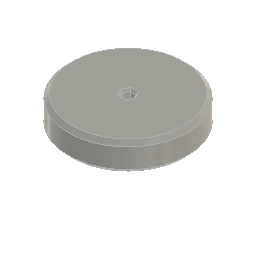
Assembly (Autodesk Fusion 360 archive; units mm, degrees)
design "Flywheel"
Autodesk Fusion 360 part; units mm, degrees
(part 1 of 2)
sketch "Sketch1" plane through (0, 0, 0) normal (0, 0, 1) x (1, 0, 0)
  circle A0 centre (0, 0) radius 2.5
  line L0 (1.3856, 0) -> (0.6928, 1.2)
  line L1 (0.6928, 1.2) -> (-0.6928, 1.2)
  line L2 (-0.6928, 1.2) -> (-1.3856, 0)
  line L3 (-1.3856, 0) -> (-0.6928, -1.2)
  line L4 (-0.6928, -1.2) -> (0.6928, -1.2)
  line L5 (0.6928, -1.2) -> (1.3856, 0)
  dimension "d2" = 5
  dimension "d11" = 2.4
  constraint coincident A0.centre origin
  constraint horizontal L1
  measures "d2" diameter of A0
  measures "d11" distance of L0 L3
extrude "Extrude1" add sketch "Sketch1" along normal blind 8
sketch "Sketch2" plane through (0, 0, 8) normal (0, 0, 1) x (-1, 0, 0)
  circle A0 centre (0, 0) radius 2.5
  circle A1 centre (0, 0) radius 15
  line L0 (-1.3856, 0) -> (-0.6928, 1.2)
  line L1 (-0.6928, 1.2) -> (0.6928, 1.2)
  line L2 (0.6928, 1.2) -> (1.3856, 0)
  line L3 (1.3856, 0) -> (0.6928, -1.2)
  line L4 (0.6928, -1.2) -> (-0.6928, -1.2)
  line L5 (-0.6928, -1.2) -> (-1.3856, 0)
  line L6 (0.6928, -1.2) -> (1.3856, 0)
  line L7 (1.3856, 0) -> (0.6928, 1.2)
  line L8 (0.6928, 1.2) -> (-0.6928, 1.2)
  line L9 (-0.6928, 1.2) -> (-1.3856, 0)
  line L10 (-1.3856, 0) -> (-0.6928, -1.2)
  line L11 (-0.6928, -1.2) -> (0.6928, -1.2)
  dimension "d5" = 30
  dimension "d12" = 2.4
  constraint coincident A0.centre A1.centre
  constraint horizontal L11
  measures "d5" diameter of A1
  measures "d12" distance of L8 L11
extrude "Extrude2" add sketch "Sketch2" along normal blind 7 contours A0 | A1
chamfer "Chamfer1" distance 0.5 angle 45 6 edges at (-1.0392, 0.6, 15) (-1.0392, -0.6, 15) (0, -1.2, 15) (1.0392, -0.6, 15) (1.0392, 0.6, 15) (0, 1.2, 15)
chamfer "Chamfer2" distance 1 angle 45 3 edges at (-2.3308, -0.904, 8) (13.9849, 5.4242, 8) (13.9849, 5.4242, 15)
chamfer "Chamfer3" distance 0.5 angle 45 6 edges at (1.0392, 0.6, 0) (0, 1.2, 0) (-1.0392, 0.6, 0) (-1.0392, -0.6, 0) (0, -1.2, 0) (1.0392, -0.6, 0)

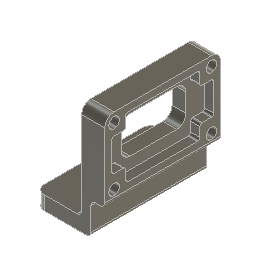
design "RPI Cam Mount"
Autodesk Fusion 360 part; units mm, degrees
sketch "Sketch1" plane through (0, 0, 0) normal (0, 0, 1) x (1, 0, 0)
  line L0 (0, 0) -> (-15, 0)
  line L1 (-15, 0) -> (-15, -25)
  line L2 (-15, -25) -> (0, -25)
  line L3 (0, -25) -> (0, 0)
  dimension "d1" = 15
  dimension "d2" = 25
  constraint horizontal L0
  constraint vertical L1
  constraint horizontal L2
  constraint vertical L3
  constraint coincident L0.start L3.end
  measures "d1" distance of L0.start L0.end
  measures "d2" distance of L0.end L1.end
extrude "Extrude1" add sketch "Sketch1" along normal blind 3
sketch "Sketch2" plane through (0, 0, 3) normal (0, 0, 1) x (-1, 0, 0)
  line L0 (0, 25) -> (0, 0)
  line L1 (0, 0) -> (15, 0)
  line L2 (15, 0) -> (15, 25)
  line L3 (15, 25) -> (0, 25)
  line L4 (0, 0) -> (5, 0)
  line L5 (5, 0) -> (5, 25)
  line L6 (5, 25) -> (0, 25)
  line L7 (0, 25) -> (0, 0)
  dimension "d5" = 5
  constraint horizontal L4
  constraint vertical L5
  constraint horizontal L6
  constraint vertical L7
  constraint coincident L3 L5.end
  constraint coincident L0.end L1.start
  measures "d5" distance of L0.end L4.end
extrude "Extrude2" add sketch "Sketch2" along normal blind 21 contours L0 L1 L3 L4 L5 L6 L7
sketch "Sketch3" plane through (0, 0, 0) normal (1, 0, 0) x (0, 1, 0)
  line L0 (-25, 0) -> (0, 0)
  line L1 (0, 0) -> (0, 24)
  line L2 (0, 24) -> (-25, 24)
  line L3 (-25, 24) -> (-25, 0)
  circle A0 centre (-23, 9.5) radius 1.15
  circle A1 centre (-23, 22) radius 1.15
  circle A2 centre (-2, 22) radius 1.15
  circle A3 centre (-2, 9.5) radius 1.15
  dimension "d8" = 2.3
  dimension "d9" = 2.3
  dimension "d10" = 2.3
  dimension "d11" = 2.3
  dimension "d12" = 14.5
  dimension "d13" = 2
  dimension "d14" = 2
  dimension "d15" = 2
  constraint vertical A0.centre A1.centre
  constraint horizontal A1.centre A2.centre
  constraint horizontal A0.centre A3.centre
  constraint vertical A2.centre A3.centre
  measures "d8" diameter of A0
  measures "d9" diameter of A1
  measures "d10" diameter of A2
  measures "d11" diameter of A3
  measures "d12" distance of L2 A3.centre
  measures "d13" distance of L2 A2.centre
  measures "d14" distance of L1 A2.centre
  measures "d15" distance of L3 A1.centre
extrude "Extrude3" cut sketch "Sketch3" against normal up to surface (5 mm away) contours A0 | A1 | A2 | A3
fillet "Fillet1" radius 2 2 edges at (-2.5, -25, 24) (-2.5, 0, 24)
sketch "Sketch4" plane through (0, -25, 0) normal (0, -1, 0) x (1, 0, 0)
  line L0 (-15, 0) -> (0, 0)
  line L1 (0, 0) -> (0, 22)
  line L2 (-5, 3) -> (-15, 3)
  line L3 (-15, 3) -> (-15, 0)
  line L4 (0, 0) -> (-3, 0)
  line L5 (-3, 0) -> (-3, 7)
  line L6 (-3, 7) -> (0, 7)
  line L7 (0, 7) -> (0, 0)
  line L8 (0, 22) -> (-5, 22)
  line L9 (-5, 22) -> (-5, 3)
  dimension "d20" = 3
  dimension "d22" = 7
  constraint horizontal L4
  constraint vertical L5
  constraint horizontal L6
  constraint vertical L7
  constraint coincident L0.end L1.start
  measures "d20" distance of L5.end L6.end
  measures "d22" distance of L4 L6
extrude "Extrude4" cut sketch "Sketch4" against normal up to surface (25 mm away) contours L0 L1 L4 L5 L6 L7
fillet "Fillet2" radius 1 1 edges at (-3, -12.5, 7)
fillet "Fillet3" radius 1 1 edges at (0, -12.5, 7)
sketch "Sketch5" plane through (0, 0, 3) normal (0, 0, 1) x (-1, 0, 0)
  line L0 (5, 25) -> (5, 0)
  line L1 (5, 0) -> (15, 0)
  line L2 (15, 0) -> (15, 25)
  line L3 (15, 25) -> (5, 25)
  circle A0 centre (9.6576, 15.5) radius 2
  circle A1 centre (9.6576, 9.5) radius 2
  line L4 (9.6576, 15.5) -> (9.6576, 9.5) construction
  line L5 (9.9151, 25) -> (9.4, 0) construction
  dimension "d29" = 4
  dimension "d30" = 4
  dimension "d31" = 6
  dimension "d32" = 9.4
  constraint vertical A0.centre A1.centre
  constraint coincident A0.centre L4.start
  constraint coincident A1.centre L4.end
  constraint midpoint L4 L5
  constraint coincident L1 L5.end
  constraint coincident L3 L5.start
  measures "d29" diameter of A1
  measures "d30" diameter of A0
  measures "d31" distance of A0.centre A1.centre
  measures "d32" distance of origin L5.end
extrude "Extrude5" cut sketch "Sketch5" against normal up to surface (3 mm away) contours A0 | A1
sketch "Sketch6" plane through (0, 0, 0) normal (1, 0, 0) x (0, 1, 0)
  line L0 (-25, 8) -> (0, 8)
  line L1 (0, 8) -> (0, 22)
  arc A0 (0, 22) -> (-2, 24) centre (-2, 22) ccw
  line L2 (-2, 24) -> (-23, 24)
  arc A1 (-23, 24) -> (-25, 22) centre (-23, 22) ccw
  line L3 (-25, 22) -> (-25, 8)
  circle A2 centre (-2, 22) radius 1.15
  circle A3 centre (-23, 22) radius 1.15
  circle A4 centre (-2, 9.5) radius 1.15
  circle A5 centre (-23, 9.5) radius 1.15
  line L4 (-7.5, 12) -> (-17.5, 12)
  line L5 (-19.5, 14) -> (-19.5, 18)
  line L6 (-17.5, 20) -> (-7.5, 20)
  line L7 (-5.5, 18) -> (-5.5, 14)
  line L8 (-5.5, 12) -> (-19.5, 20) construction
  line L9 (-19.5, 12) -> (-5.5, 20) construction
  line L10 (-12.5, 24) -> (-12.5, 8) construction
  line L11 (-12.5, 16) -> (0, 16) construction
  arc A6 (-17.5, 20) -> (-19.5, 18) centre (-17.5, 18) ccw
  arc A7 (-5.5, 18) -> (-7.5, 20) centre (-7.5, 18) ccw
  arc A8 (-7.5, 12) -> (-5.5, 14) centre (-7.5, 14) ccw
  arc A9 (-19.5, 14) -> (-17.5, 12) centre (-17.5, 14) ccw
  point P0 (-12.5, 16)
  dimension "d41" = 14
  dimension "d42" = 8
  dimension "d43" = 2
  constraint horizontal L4
  constraint perpendicular L4 L5
  constraint parallel L4 L6
  constraint parallel L5 L7
  constraint coincident L8 P0
  constraint coincident L9 P0
  constraint midpoint L2 L10.start
  constraint midpoint L0 L10.end
  constraint midpoint L10 P0
  constraint coincident L1 L11.end
  constraint perpendicular L1 L11
  constraint coincident P0 L11.start
  constraint coincident L8.end L5
  constraint coincident L8.end L6
  constraint tangent L5 A6
  constraint tangent L6 A6
  constraint coincident L9.end L7
  constraint coincident L9.end L6
  constraint tangent L7 A7
  constraint tangent L6 A7
  constraint equal A6 A7
  constraint coincident L8.start L4
  constraint coincident L8.start L7
  constraint tangent L4 A8
  constraint tangent L7 A8
  constraint equal A6 A8
  constraint coincident L9.start L4
  constraint coincident L9.start L5
  constraint tangent L4 A9
  constraint tangent L5 A9
  constraint equal A6 A9
  measures "d41" distance of L8.end L9.end
  measures "d42" distance of L8.start L9.end
  measures "d43" radius of A6
fillet "Fillet4" radius 1 1 edges at (-5, -12.5, 3)
fillet "Fillet5" radius 2 2 edges at (-15, -25, 1.5) (-15, 0, 1.5)
fillet "Fillet6" radius 1 1 edges at (-3, -12.5, 0)
extrude "Extrude6" cut sketch "Sketch6" against normal up to surface (5 mm away) contours L4 L5 L6 L7 A6 A7 A8 A9
sketch "Sketch7" plane through (0, 0, 0) normal (1, 0, 0) x (0, 1, 0)
  line L0 (-5.5, 18) -> (-5.5, 14)
  arc A0 (-7.5, 12) -> (-5.5, 14) centre (-7.5, 14) ccw
  line L1 (-7.5, 12) -> (-17.5, 12)
  arc A1 (-19.5, 14) -> (-17.5, 12) centre (-17.5, 14) ccw
  line L2 (-19.5, 14) -> (-19.5, 18)
  arc A2 (-17.5, 20) -> (-19.5, 18) centre (-17.5, 18) ccw
  line L3 (-17.5, 20) -> (-7.5, 20)
  arc A3 (-5.5, 18) -> (-7.5, 20) centre (-7.5, 18) ccw
  line L4 (-25, 8) -> (0, 8)
  line L5 (0, 8) -> (0, 22)
  arc A4 (0, 22) -> (-2, 24) centre (-2, 22) ccw
  line L6 (-2, 24) -> (-23, 24)
  arc A5 (-23, 24) -> (-25, 22) centre (-23, 22) ccw
  line L7 (-25, 22) -> (-25, 8)
  circle A6 centre (-2, 22) radius 1.15
  circle A7 centre (-23, 22) radius 1.15
  circle A8 centre (-2, 9.5) radius 1.15
  circle A9 centre (-23, 9.5) radius 1.15
  line L8 (-23.5, 13) -> (-23.5, 19)
  line L9 (-23, 19.5) -> (-21, 19.5)
  line L10 (-20.5, 20) -> (-20.5, 22)
  line L11 (-20, 22.5) -> (-5, 22.5)
  line L12 (-4.5, 22) -> (-4.5, 20)
  line L13 (-4, 19.5) -> (-2, 19.5)
  line L14 (-1.5, 19) -> (-1.5, 13)
  line L15 (-2, 12.5) -> (-4, 12.5)
  line L16 (-4.5, 12) -> (-4.5, 10)
  line L17 (-5, 9.5) -> (-20, 9.5)
  line L18 (-20.5, 10) -> (-20.5, 12)
  line L19 (-21, 12.5) -> (-23, 12.5)
  arc A10 (-23, 19.5) -> (-23.5, 19) centre (-23, 19) ccw
  arc A11 (-21, 19.5) -> (-20.5, 20) centre (-21, 20) ccw
  arc A12 (-20, 22.5) -> (-20.5, 22) centre (-20, 22) ccw
  arc A13 (-4.5, 22) -> (-5, 22.5) centre (-5, 22) ccw
  arc A14 (-4.5, 20) -> (-4, 19.5) centre (-4, 20) ccw
  arc A15 (-1.5, 19) -> (-2, 19.5) centre (-2, 19) ccw
  arc A16 (-2, 12.5) -> (-1.5, 13) centre (-2, 13) ccw
  arc A17 (-4, 12.5) -> (-4.5, 12) centre (-4, 12) ccw
  arc A18 (-5, 9.5) -> (-4.5, 10) centre (-5, 10) ccw
  arc A19 (-20.5, 10) -> (-20, 9.5) centre (-20, 10) ccw
  arc A20 (-20.5, 12) -> (-21, 12.5) centre (-21, 12) ccw
  arc A21 (-23.5, 13) -> (-23, 12.5) centre (-23, 13) ccw
  point P0 (-23.5, 19.5)
  point P1 (-20.5, 19.5)
  point P2 (-20.5, 22.5)
  dimension "d46" = 3
  dimension "d47" = 3
  dimension "d48" = 1.5
  dimension "d49" = 1.5
  dimension "d50" = 1.5
  dimension "d51" = 1.5
  dimension "d52" = 0.5
  constraint perpendicular L6 L8
  constraint perpendicular L8 L9
  constraint perpendicular L9 L10
  constraint perpendicular L10 L11
  constraint perpendicular L11 L12
  constraint perpendicular L12 L13
  constraint perpendicular L13 L14
  constraint perpendicular L14 L15
  constraint perpendicular L13 L16
  constraint perpendicular L16 L17
  constraint perpendicular L17 L18
  constraint perpendicular L8 L19
  constraint coincident P0 L8
  constraint coincident P0 L9
  constraint tangent L8 A10
  constraint tangent L9 A10
  constraint coincident P1 L9
  constraint coincident P1 L10
  constraint tangent L9 A11
  constraint tangent L10 A11
  constraint equal A10 A11
  constraint coincident P2 L10
  constraint coincident P2 L11
  constraint tangent L10 A12
  constraint tangent L11 A12
  constraint equal A10 A12
  constraint tangent L11 A13
  constraint tangent L12 A13
  constraint equal A10 A13
  constraint tangent L12 A14
  constraint tangent L13 A14
  constraint equal A10 A14
  constraint tangent L13 A15
  constraint tangent L14 A15
  constraint equal A10 A15
  constraint tangent L14 A16
  constraint tangent L15 A16
  constraint equal A10 A16
  constraint tangent L15 A17
  constraint tangent L16 A17
  constraint equal A10 A17
  constraint tangent L16 A18
  constraint tangent L17 A18
  constraint equal A10 A18
  constraint tangent L17 A19
  constraint tangent L18 A19
  constraint equal A10 A19
  constraint tangent L18 A20
  constraint tangent L19 A20
  constraint equal A10 A20
  constraint tangent L8 A21
  constraint tangent L19 A21
  constraint equal A10 A21
  measures "d46" distance of P0 P1
  measures "d47" distance of P1 P2
  measures "d48" distance of L7 L8
  measures "d49" distance of L5 L14
  measures "d50" distance of L4 L17
  measures "d51" distance of L6 L11
  measures "d52" radius of A10
extrude "Extrude7" cut sketch "Sketch7" against normal blind 2 contours L8 L9 L10 L11 L12 L13 L14 L15 L16 L17 L18 L19 A10 A11 A12 A13 A14 A15 A16 A17 A18 A19 A20 A21

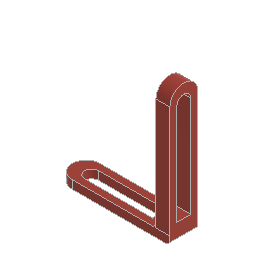
design "General Mount"
Autodesk Fusion 360 part; units mm, degrees
sketch "Sketch1" plane through (0, 0, 0) normal (0, 0, 1) x (1, 0, 0)
  line L0 (17.5, -5) -> (-17.5, -5)
  line L1 (-17.5, -5) -> (-17.5, 5)
  line L2 (-17.5, 5) -> (17.5, 5)
  line L3 (17.5, 5) -> (17.5, -5)
  line L4 (17.5, -5) -> (-17.5, 5) construction
  line L5 (-17.5, -5) -> (17.5, 5) construction
  circle A0 centre (-17.5, 0) radius 5
  line L6 (8.75, -2.5) -> (-15.5, -2.5)
  line L7 (-15.5, -2.5) -> (-15.5, 2.5)
  line L8 (-15.5, 2.5) -> (8.75, 2.5)
  line L9 (8.75, 2.5) -> (8.75, -2.5)
  line L10 (8.75, -2.5) -> (-7.151, 2.0431) construction
  circle A1 centre (-15.5, 0) radius 2.5
  dimension "d1" = 35
  dimension "d2" = 10
  dimension "d3" = 5
  dimension "d17" = 2
  constraint horizontal L0
  constraint perpendicular L0 L1
  constraint parallel L0 L2
  constraint parallel L1 L3
  constraint coincident L4 origin
  constraint coincident L5 origin
  constraint midpoint L1 A0.centre
  constraint coincident L0.end A0
  constraint horizontal L6
  constraint perpendicular L6 L7
  constraint parallel L6 L8
  constraint parallel L7 L9
  constraint coincident L10 origin
  constraint coincident L4 L6.start
  constraint midpoint L7 A1.centre
  constraint coincident L6.end A1
  constraint horizontal origin A1.centre
  constraint coincident L7.end L8.start
  constraint coincident L6.end L7.start
  measures "d1" distance of L1.end L2.end
  measures "d2" distance of L0.start L2.end
  measures "d3" distance of L6.start L8.end
  measures "d17" distance of L1 L7
extrude "Extrude1" add sketch "Sketch1" along normal blind 3 contours L0 L2 L3 A0 L6 L8 L9 | L1 A0 A1 | L1 A0 L6 A1 | L1 A0 L8 A1
sketch "Sketch2" plane through (0, 0, 3) normal (0, 0, 1) x (-1, 0, 0)
  arc A0 (15.5, -2.5) -> (15.5, 2.5) centre (15.5, 0) ccw
  line L0 (15.5, -2.5) -> (-8.75, -2.5)
  line L1 (-8.75, -2.5) -> (-8.75, 2.5)
  line L2 (-8.75, 2.5) -> (15.5, 2.5)
  arc A1 (17.5, -5) -> (17.5, 5) centre (17.5, 0) ccw
  line L3 (17.5, 5) -> (-17.5, 5)
  line L4 (-17.5, 5) -> (-17.5, -5)
  line L5 (-17.5, -5) -> (17.5, -5)
  line L6 (-17.5, -5) -> (-12.5, -5)
  line L7 (-12.5, -5) -> (-12.5, 5)
  line L8 (-12.5, 5) -> (-17.5, 5)
  line L9 (-17.5, 5) -> (-17.5, -5)
  dimension "d6" = 5
  constraint horizontal L6
  constraint vertical L7
  constraint horizontal L8
  constraint vertical L9
  constraint coincident L3 L7.end
  constraint coincident L4.end L5.start
  measures "d6" distance of L4.end L6.end
extrude "Extrude2" add sketch "Sketch2" along normal blind 45 contours L3 L4 L5 L6 L7 L8 L9
sketch "Sketch3" plane through (17.5, 0, 0) normal (1, 0, 0) x (0, 1, 0)
  line L0 (-5, 0) -> (5, 0)
  line L1 (5, 0) -> (5, 48)
  line L2 (5, 48) -> (-5, 48)
  line L3 (-5, 48) -> (-5, 3)
  line L4 (-5, 3) -> (-5, 0)
  circle A0 centre (0, 43) radius 5
  line L5 (2.5, 6) -> (-2.5, 6)
  line L6 (-2.5, 6) -> (-2.5, 42)
  line L7 (-2.5, 42) -> (2.5, 42)
  line L8 (2.5, 42) -> (2.5, 6)
  circle A1 centre (0, 42) radius 2.5
  dimension "d9" = 5
  dimension "d10" = 2.5
  dimension "d11" = 6
  dimension "d12" = 6
  constraint tangent L1 A0
  constraint tangent L2 A0
  constraint tangent L3 A0
  constraint horizontal L5
  constraint vertical L6
  constraint horizontal L7
  constraint vertical L8
  constraint midpoint L7 A1.centre
  constraint coincident L7.end A1
  measures "d9" distance of L5.start L5.end
  measures "d10" distance of L1 L8
  measures "d11" distance of L0 L5
  measures "d12" distance of L2 L7
extrude "Extrude3" cut sketch "Sketch3" against normal blind 10 contours L1 L2 A0 | L2 L3 A0 | A0 L5 L6 L8 | A0 L6 L8 A1 | L7 A1 | L7 A1 picked at (1.8589, 38.9501)
chamfer "Chamfer2" distance 1 angle 45 2 edges at (17.5, 0, 0) (12.5, 0, 3)
sketch "Sketch4" plane through (0, 0, 3) normal (0, 0, 1) x (-1, 0, 0)
  line L0 (-11.5, 5) -> (-11.5, -5)
  line L1 (-11.5, -5) -> (17.5, -5)
  arc A0 (17.5, -5) -> (17.5, 5) centre (17.5, 0) ccw
  line L2 (17.5, 5) -> (-11.5, 5)
  arc A1 (15.5, -2.5) -> (15.5, 2.5) centre (15.5, 0) ccw
  line L3 (15.5, -2.5) -> (-8.75, -2.5)
  line L4 (-8.75, -2.5) -> (-8.75, 2.5)
  line L5 (-8.75, 2.5) -> (15.5, 2.5)
  line L6 (20.7, -1) -> (20.7, 1)
  line L7 (20.7, 1) -> (18.9679, 0)
  line L8 (18.9679, 0) -> (20.7, -1)
  dimension "d18" = 60
  dimension "d19" = 60
  dimension "d20" = 2
  dimension "d21" = 3.2
  constraint vertical L6
  constraint horizontal origin L7.end
  measures "d18" angle of L6 L7
  measures "d19" angle of L6 L8
  measures "d20" distance of L6.start L6.end
  measures "d21" distance of A0.centre L6
sketch "Sketch5" plane through (12.5, 0, 0) normal (-1, 0, 0) x (0, -1, 0)
  arc A0 (2.5, 42) -> (-2.5, 42) centre (0, 42) ccw
  line L0 (2.5, 42) -> (2.5, 6)
  line L1 (2.5, 6) -> (-2.5, 6)
  line L2 (-2.5, 6) -> (-2.5, 42)
  line L3 (-5, 4) -> (5, 4)
  line L4 (5, 4) -> (5, 43)
  arc A1 (5, 43) -> (-5, 43) centre (0, 43) ccw
  line L5 (-5, 43) -> (-5, 4)
  line L6 (-1, 47) -> (1, 47)
  line L7 (1, 47) -> (0, 45.2679)
  line L8 (0, 45.2679) -> (-1, 47)
  dimension "d22" = 60
  dimension "d23" = 60
  dimension "d24" = 2
  dimension "d25" = 4
  constraint perpendicular L2 L6
  constraint vertical origin L7.end
  measures "d22" angle of L6 L8
  measures "d23" angle of L6 L7
  measures "d24" distance of L6.start L6.end
  measures "d25" distance of A1.centre L6
loft "Loft1" [rolled back]
fillet "Fillet1" [rolled back] radius 0.1

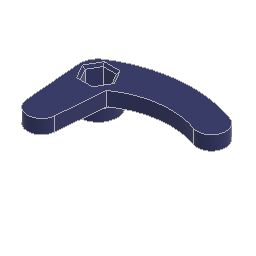
design "Servo Arm"
Autodesk Fusion 360 part; units mm, degrees
sketch "Sketch1" plane through (0, 0, 0) normal (0, 0, 1) x (1, 0, 0)
  circle A0 centre (0, 0) radius 2.425
  circle A1 centre (0, 0) radius 4
  line L0 (-3.9861, -0.3333) -> (-2.9896, -12.25)
  line L1 (3.9861, -0.3333) -> (2.9896, -12.25)
  circle A2 centre (0, -12) radius 3
  circle A3 centre (21, 3) radius 3
  circle A4 centre (12.4213, -19.949) radius 27.5
  circle A5 centre (14.1277, -16.755) radius 17.9162
  line L2 (-1.4001, 2.425) -> (-2.8001, 0)
  line L3 (-2.8001, 0) -> (-1.4001, -2.425)
  line L4 (-1.4001, -2.425) -> (1.4001, -2.425)
  line L5 (1.4001, -2.425) -> (2.8001, 0)
  line L6 (2.8001, 0) -> (1.4001, 2.425)
  line L7 (1.4001, 2.425) -> (-1.4001, 2.425)
  dimension "d1" = 4.85
  dimension "d2" = 8
  dimension "d3" = 6
  dimension "d4" = 12
  dimension "d5" = 6
  dimension "d6" = 55
  constraint coincident A0.centre A1.centre
  constraint concentric A0 A1
  constraint coincident A1 L0.start
  constraint coincident A1 L1.start
  constraint tangent A1 L1
  constraint tangent A1 L0
  constraint vertical A0.centre A2.centre
  constraint tangent L1 A2
  constraint tangent L0 A2
  constraint coincident L1.end A2
  constraint coincident L0.end A2
  constraint tangent A1 A4
  constraint tangent A3 A4
  constraint tangent A1 A5
  constraint tangent A3 A5
  constraint horizontal L4
  constraint tangent A0 L4
  measures "d1" diameter of A0
  measures "d2" diameter of A1
  measures "d3" diameter of A2
  measures "d4" distance of A0.centre A2.centre
  measures "d5" diameter of A3
  measures "d6" diameter of A4
extrude "Extrude1" add sketch "Sketch1" along normal blind 3 contours A1 | A1 L1 A5 | A1 L1 A3 A4 A5 | A1 L0 A5 | L0 L1 A2 A5 | A2 | A3 picked at (1.496, -7.129)
sketch "Sketch2" plane through (0, 0, 0) normal (0, 0, -1) x (1, 0, 0)
  arc A0 (22.0505, -5.8101) -> (20.0143, -0.1666) centre (21, -3) ccw
  arc A1 (3.8394, 2.0872) -> (20.0143, -0.1666) centre (14.1277, 16.755) ccw
  line L0 (3.8394, 2.0872) -> (2.9896, 12.25)
  arc A2 (2.9896, 12.25) -> (-2.9896, 12.25) centre (0, 12) ccw
  line L1 (-2.9896, 12.25) -> (-3.9861, 0.3333)
  arc A3 (-3.9861, 0.3333) -> (-2.1143, -3.3956) centre (0, 0) ccw
  arc A4 (-2.1143, -3.3956) -> (22.0505, -5.8101) centre (12.4213, 19.949) ccw
  circle A5 centre (0, 0) radius 4
  line L2 (1.4001, -2.425) -> (-1.4001, -2.425)
  line L3 (-1.4001, -2.425) -> (-2.8001, 0)
  line L4 (-2.8001, 0) -> (-1.4001, 2.425)
  line L5 (-1.4001, 2.425) -> (1.4001, 2.425)
  line L6 (1.4001, 2.425) -> (2.8001, 0)
  line L7 (2.8001, 0) -> (1.4001, -2.425)
  line L8 (1.4001, -2.425) -> (2.8001, 0)
  line L9 (2.8001, 0) -> (1.4001, 2.425)
  line L10 (1.4001, 2.425) -> (-1.4001, 2.425)
  line L11 (-1.4001, 2.425) -> (-2.8001, 0)
  line L12 (-2.8001, 0) -> (-1.4001, -2.425)
  line L13 (-1.4001, -2.425) -> (1.4001, -2.425)
  dimension "d11" = 8
  dimension "d12" = 4.85
  constraint coincident A3.centre A5.centre
  constraint horizontal L10
  measures "d11" diameter of A5
  measures "d12" distance of L10 L13
extrude "Extrude2" add sketch "Sketch2" along normal blind 3 contours A3 A5
chamfer "Chamfer3" distance 0.5 angle 45 13 edges at (3.5749, -1.7945, 0) (0, -2.425, -3) (-2.1001, -1.2125, -3) (-2.1001, 1.2125, -3) (0, 2.425, -3) (2.1001, 1.2125, -3) (2.1001, -1.2125, -3) (0, 2.425, 3) (-2.1001, 1.2125, 3) (-2.1001, -1.2125, 3) (0, -2.425, 3) (2.1001, -1.2125, 3) (2.1001, 1.2125, 3)

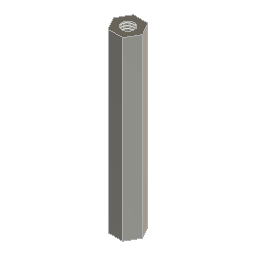
design "Pillar 35mm"
Autodesk Fusion 360 part; units mm, degrees
sketch "Sketch1" plane through (0, 0, 0) normal (0, 0, 1) x (1, 0, 0)
  line L0 (-1.4434, 2.5) -> (-2.8868, 0)
  line L1 (-2.8868, 0) -> (-1.4434, -2.5)
  line L2 (-1.4434, -2.5) -> (1.4434, -2.5)
  line L3 (1.4434, -2.5) -> (2.8868, 0)
  line L4 (2.8868, 0) -> (1.4434, 2.5)
  line L5 (1.4434, 2.5) -> (-1.4434, 2.5)
  dimension "d1" = 5
  measures "d1" distance of L0 L3
extrude "Extrude1" add sketch "Sketch1" along normal blind 35
sketch "Sketch2" plane through (0, 0, 35) normal (0, 0, 1) x (-1, 0, 0)
  line L0 (-1.4434, -2.5) -> (1.4434, -2.5)
  line L1 (1.4434, -2.5) -> (2.8868, 0)
  line L2 (2.8868, 0) -> (1.4434, 2.5)
  line L3 (1.4434, 2.5) -> (-1.4434, 2.5)
  line L4 (-1.4434, 2.5) -> (-2.8868, 0)
  line L5 (-2.8868, 0) -> (-1.4434, -2.5)
  circle A0 centre (0, 0) radius 1.5
  dimension "d4" = 3
  constraint coincident A0.centre origin
  measures "d4" diameter of A0
extrude "Extrude2" cut sketch "Sketch2" against normal blind 8 contours A0
sketch "Sketch3" plane through (0, 0, 0) normal (0, 0, -1) x (1, 0, 0)
  line L0 (-1.4434, -2.5) -> (1.4434, -2.5)
  line L1 (1.4434, -2.5) -> (2.8868, 0)
  line L2 (2.8868, 0) -> (1.4434, 2.5)
  line L3 (1.4434, 2.5) -> (-1.4434, 2.5)
  line L4 (-1.4434, 2.5) -> (-2.8868, 0)
  line L5 (-2.8868, 0) -> (-1.4434, -2.5)
  circle A0 centre (0, 0) radius 1.5
  dimension "d7" = 3
  constraint coincident A0.centre origin
  measures "d7" diameter of A0
extrude "Extrude3" cut sketch "Sketch3" against normal blind 8 contours A0
thread "Thread1" "ISO Metric profile 3.0 M3x0.5 M3x0.5 6H" major diameter 3.086 minor diameter 2.529 pitch 0.5 angle 60 resizes the face on face at (1.4981, 0.0748, 5.3333) on face at (-1.4925, 0.1494, 32.3333)

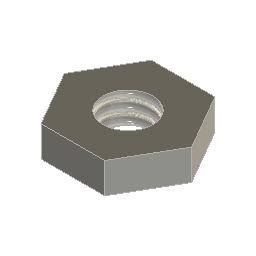
design "M2_nut"
Autodesk Fusion 360 part; units mm, degrees
sketch "Sketch1" plane through (0, 0, 0) normal (0, 0, 1) x (1, 0, 0)
  line L0 (2.0785, 0) -> (1.0392, 1.8)
  line L1 (1.0392, 1.8) -> (-1.0392, 1.8)
  line L2 (-1.0392, 1.8) -> (-2.0785, 0)
  line L3 (-2.0785, 0) -> (-1.0392, -1.8)
  line L4 (-1.0392, -1.8) -> (1.0392, -1.8)
  line L5 (1.0392, -1.8) -> (2.0785, 0)
  circle A0 centre (0, 0) radius 1
  dimension "d1" = 3.6
  dimension "d2" = 2
  constraint coincident A0.centre origin
  constraint horizontal L1
  measures "d1" distance of L0 L3
  measures "d2" diameter of A0
extrude "Extrude1" add sketch "Sketch1" along normal blind 1
thread "Thread1" "ISO Metric profile 2.0 M2x0.4 M2x0.4 6H" major diameter 2.074 minor diameter 1.623 pitch 0.4 angle 60 resizes the face on face at (0.9988, -0.0498, 0.6667)

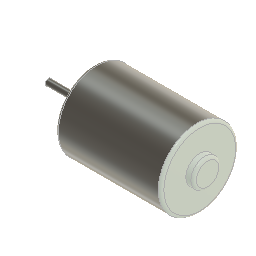
design "RS380 Manual"
Autodesk Fusion 360 part; units mm, degrees
sketch "Sketch1" plane through (0, 0, 0) normal (0, 1, 0) x (1, 0, 0)
  line L0 (0, 0) -> (35, 0) construction
  line L1 (54.2, -13.85) -> (16.4, -13.85)
  line L2 (16.4, -13.85) -> (16.4, -5)
  line L3 (16.4, -5) -> (13.8, -5)
  line L4 (13.8, -5) -> (13.8, -1.15)
  line L5 (13.8, -1.15) -> (0, -1.15)
  line L6 (0, -1.15) -> (0, 0)
  line L7 (0, 0) -> (57, 0)
  line L8 (54.2, -13.85) -> (54.2, -5)
  line L9 (54.2, -5) -> (57, -5)
  line L10 (57, -5) -> (57, 0)
  dimension "d1" = 35
  dimension "d2" = 1.15
  dimension "d3" = 13.8
  dimension "d4" = 2.6
  dimension "d5" = 5
  dimension "d6" = 13.85
  dimension "d7" = 57
  dimension "d8" = 5
  dimension "d9" = 37.8
  constraint coincident L0.start L6.end
  constraint horizontal L0
  constraint perpendicular L1 L2
  constraint perpendicular L2 L3
  constraint perpendicular L3 L4
  constraint perpendicular L4 L5
  constraint perpendicular L3 L6
  constraint coincident L0.start L7
  constraint perpendicular L1 L8
  constraint perpendicular L8 L9
  constraint perpendicular L9 L10
  constraint horizontal L7
  measures "d1" distance of L0.start L0.end
  measures "d2" distance of L5.end L0.start
  measures "d3" distance of L4.end L5.end
  measures "d4" distance of L2.end L3.end
  measures "d5" distance of L3 L7
  measures "d6" distance of L1 L7
  measures "d7" distance of L0.start L7.end
  measures "d8" distance of L9.end L7.end
  measures "d9" distance of L1.start L1.end
revolve "Revolve1" add sketch "Sketch1" angle 360 about axis through (0, 0, 0) along (1, 0, 0)
fillet "Fillet1" radius 1 4 edges at (54.2, -5.0084, -12.9127) (57, -1.8081, -4.6616) (16.4, -5.0084, -12.9127) (13.8, -1.8081, -4.6616)
equation "d2 = ( 2.3 / 2 ) * 1 mm"
equation "d3 = 16.4 mm - 2.6 mm"
equation "d6 = ( 27.7 / 2 ) * 1 mm"

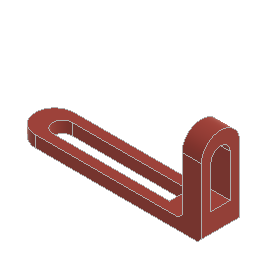
design "General Mount Short"
Autodesk Fusion 360 part; units mm, degrees
sketch "Sketch1" plane through (0, 0, 0) normal (0, 0, 1) x (1, 0, 0)
  line L0 (21.5, -5) -> (-21.5, -5)
  line L1 (-21.5, -5) -> (-21.5, 5)
  line L2 (-21.5, 5) -> (21.5, 5)
  line L3 (21.5, 5) -> (21.5, -5)
  line L4 (21.5, -5) -> (-21.5, 5) construction
  line L5 (-21.5, -5) -> (21.5, 5) construction
  circle A0 centre (-21.5, 0) radius 5
  line L6 (10.75, -2.5) -> (-19.5, -2.5)
  line L7 (-19.5, -2.5) -> (-19.5, 2.5)
  line L8 (-19.5, 2.5) -> (10.75, 2.5)
  line L9 (10.75, 2.5) -> (10.75, -2.5)
  line L10 (10.75, -2.5) -> (-7.2492, 1.6859) construction
  circle A1 centre (-19.5, 0) radius 2.5
  dimension "d1" = 43
  dimension "d2" = 10
  dimension "d3" = 5
  dimension "d17" = 2
  constraint horizontal L0
  constraint perpendicular L0 L1
  constraint parallel L0 L2
  constraint parallel L1 L3
  constraint coincident L4 origin
  constraint coincident L5 origin
  constraint midpoint L1 A0.centre
  constraint coincident L0.end A0
  constraint horizontal L6
  constraint perpendicular L6 L7
  constraint parallel L6 L8
  constraint parallel L7 L9
  constraint coincident L10 origin
  constraint coincident L4 L6.start
  constraint midpoint L7 A1.centre
  constraint coincident L6.end A1
  constraint horizontal origin A1.centre
  constraint coincident L7.end L8.start
  constraint coincident L6.end L7.start
  measures "d1" distance of L1.end L2.end
  measures "d2" distance of L0.start L2.end
  measures "d3" distance of L6.start L8.end
  measures "d17" distance of L1 L7
extrude "Extrude1" add sketch "Sketch1" along normal blind 3 contours L0 L2 L3 A0 L6 L8 L9 | L1 A0 A1 | L1 A0 L6 A1 | L1 A0 L8 A1
sketch "Sketch2" plane through (0, 0, 3) normal (0, 0, 1) x (-1, 0, 0)
  arc A0 (19.5, -2.5) -> (19.5, 2.5) centre (19.5, 0) ccw
  line L0 (19.5, -2.5) -> (-10.75, -2.5)
  line L1 (-10.75, -2.5) -> (-10.75, 2.5)
  line L2 (-10.75, 2.5) -> (19.5, 2.5)
  arc A1 (21.5, -5) -> (21.5, 5) centre (21.5, 0) ccw
  line L3 (21.5, 5) -> (-21.5, 5)
  line L4 (-21.5, 5) -> (-21.5, -5)
  line L5 (-21.5, -5) -> (21.5, -5)
  line L6 (-21.5, -5) -> (-16.5, -5)
  line L7 (-16.5, -5) -> (-16.5, 5)
  line L8 (-16.5, 5) -> (-21.5, 5)
  line L9 (-21.5, 5) -> (-21.5, -5)
  dimension "d6" = 5
  constraint horizontal L6
  constraint vertical L7
  constraint horizontal L8
  constraint vertical L9
  constraint coincident L3 L7.end
  constraint coincident L4.end L5.start
  measures "d6" distance of L4.end L6.end
extrude "Extrude2" add sketch "Sketch2" along normal blind 20 contours L3 L4 L5 L6 L7 L8 L9
sketch "Sketch3" plane through (21.5, 0, 0) normal (1, 0, 0) x (0, 1, 0)
  line L0 (-5, 0) -> (5, 0)
  line L1 (5, 0) -> (5, 23)
  line L2 (5, 23) -> (-5, 23)
  line L3 (-5, 23) -> (-5, 0)
  circle A0 centre (0, 18) radius 5
  line L4 (2.5, 6) -> (-2.5, 6)
  line L5 (-2.5, 6) -> (-2.5, 17)
  line L6 (-2.5, 17) -> (2.5, 17)
  line L7 (2.5, 17) -> (2.5, 6)
  circle A1 centre (0, 17) radius 2.5
  dimension "d9" = 5
  dimension "d10" = 2.5
  dimension "d11" = 6
  dimension "d12" = 6
  constraint tangent L1 A0
  constraint tangent L2 A0
  constraint horizontal L4
  constraint vertical L5
  constraint horizontal L6
  constraint vertical L7
  constraint midpoint L6 A1.centre
  constraint coincident L6.end A1
  measures "d9" distance of L4.start L4.end
  measures "d10" distance of L1 L7
  measures "d11" distance of L0 L4
  measures "d12" distance of L2 L6
extrude "Extrude3" cut sketch "Sketch3" against normal blind 10 contours L2 L3 A0 | L1 L2 A0 | A0 L5 L7 A1 | A0 L4 L5 L7 | L6 A1 | L6 A1 picked at (1.8589, 13.9501)
chamfer "Chamfer2" distance 1 angle 45 2 edges at (21.5, 0, 0) (16.5, 0, 3)

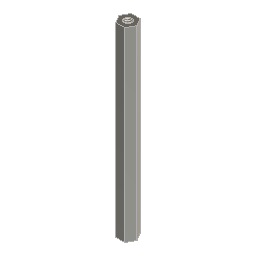
design "Pillar 60mm"
Autodesk Fusion 360 part; units mm, degrees
sketch "Sketch1" plane through (0, 0, 0) normal (0, 0, 1) x (1, 0, 0)
  line L0 (-1.4434, 2.5) -> (-2.8868, 0)
  line L1 (-2.8868, 0) -> (-1.4434, -2.5)
  line L2 (-1.4434, -2.5) -> (1.4434, -2.5)
  line L3 (1.4434, -2.5) -> (2.8868, 0)
  line L4 (2.8868, 0) -> (1.4434, 2.5)
  line L5 (1.4434, 2.5) -> (-1.4434, 2.5)
  dimension "d1" = 5
  measures "d1" distance of L0 L3
extrude "Extrude1" add sketch "Sketch1" along normal blind 60
sketch "Sketch2" plane through (0, 0, 60) normal (0, 0, 1) x (-1, 0, 0)
  line L0 (-1.4434, -2.5) -> (1.4434, -2.5)
  line L1 (1.4434, -2.5) -> (2.8868, 0)
  line L2 (2.8868, 0) -> (1.4434, 2.5)
  line L3 (1.4434, 2.5) -> (-1.4434, 2.5)
  line L4 (-1.4434, 2.5) -> (-2.8868, 0)
  line L5 (-2.8868, 0) -> (-1.4434, -2.5)
  circle A0 centre (0, 0) radius 1.5
  dimension "d4" = 3
  constraint coincident A0.centre origin
  measures "d4" diameter of A0
extrude "Extrude2" cut sketch "Sketch2" against normal blind 8 contours A0
sketch "Sketch3" plane through (0, 0, 0) normal (0, 0, -1) x (1, 0, 0)
  line L0 (-1.4434, -2.5) -> (1.4434, -2.5)
  line L1 (1.4434, -2.5) -> (2.8868, 0)
  line L2 (2.8868, 0) -> (1.4434, 2.5)
  line L3 (1.4434, 2.5) -> (-1.4434, 2.5)
  line L4 (-1.4434, 2.5) -> (-2.8868, 0)
  line L5 (-2.8868, 0) -> (-1.4434, -2.5)
  circle A0 centre (0, 0) radius 1.5
  dimension "d7" = 3
  constraint coincident A0.centre origin
  measures "d7" diameter of A0
extrude "Extrude3" cut sketch "Sketch3" against normal blind 8 contours A0
thread "Thread1" "ISO Metric profile 3.0 M3x0.5 M3x0.5 6H" major diameter 3.086 minor diameter 2.529 pitch 0.5 angle 60 resizes the face on face at (1.4981, 0.0748, 5.3333) on face at (-1.4925, 0.1494, 57.3333)

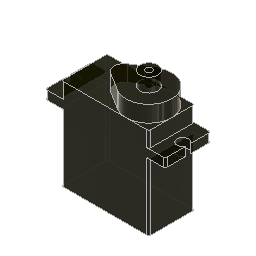
design "MG90S Servo"
Autodesk Fusion 360 part; units mm, degrees
sketch "Sketch1" plane through (0, 0, 0) normal (0, 0, 1) x (1, 0, 0)
  line L0 (11.5, 6) -> (-11.5, 6)
  line L1 (-11.5, 6) -> (-11.5, -6)
  line L2 (-11.5, -6) -> (11.5, -6)
  line L3 (11.5, -6) -> (11.5, 6)
  line L4 (11.5, 6) -> (-11.5, -6) construction
  line L5 (-11.5, 6) -> (11.5, -6) construction
  dimension "d1" = 23
  dimension "d2" = 12
  constraint horizontal L0
  constraint perpendicular L0 L1
  constraint parallel L0 L2
  constraint parallel L1 L3
  constraint coincident L4 origin
  constraint coincident L5 origin
  measures "d1" distance of L0.start L0.end
  measures "d2" distance of L0.start L2.end
extrude "Extrude1" add sketch "Sketch1" along normal blind 24.1
sketch "Sketch2" plane through (0, 0, 24.1) normal (0, 0, 1) x (-1, 0, 0)
  line L0 (-11.5, 6) -> (-11.5, -6)
  line L1 (-11.5, -6) -> (11.5, -6)
  line L2 (11.5, -6) -> (11.5, 6)
  line L3 (11.5, 6) -> (-11.5, 6)
  circle A0 centre (-5.5, 0) radius 6
  circle A1 centre (1, 0) radius 2.6
  line L4 (2.36, -2.2159) -> (-2.3615, -5.1137)
  line L5 (-2.3615, 5.1137) -> (2.36, 2.2159)
  dimension "d5" = 5.2
  dimension "d6" = 1
  constraint tangent L1 A0
  constraint tangent L0 A0
  constraint tangent L3 A0
  constraint horizontal origin A1.centre
  constraint coincident A1 L4.start
  constraint coincident A0 L4.end
  constraint coincident A0 L5.start
  constraint coincident A1 L5.end
  constraint tangent A0 L4
  constraint tangent A1 L4
  constraint tangent A1 L5
  constraint tangent A0 L5
  measures "d5" diameter of A1
  measures "d6" distance of origin A1.centre
extrude "Extrude2" add sketch "Sketch2" along normal blind 4.3 contours A0 A1 | A0 A1 L5 | A0 A1 L4 | A0 A1 | A0 A1
sketch "Sketch3" plane through (0, 0, 28.4) normal (0, 0, 1) x (-1, 0, 0)
  arc A0 (2.36, -2.2159) -> (2.36, 2.2159) centre (1, 0) ccw
  line L0 (2.36, 2.2159) -> (-2.3615, 5.1137)
  arc A1 (-2.3615, 5.1137) -> (-2.3615, -5.1137) centre (-5.5, 0) ccw
  line L1 (-2.3615, -5.1137) -> (2.36, -2.2159)
  circle A2 centre (-5.5, 0) radius 2.35
  circle A3 centre (-5.5, 0) radius 0.85
  dimension "d9" = 4.7
  dimension "d12" = 1.5
  constraint concentric A1 A2
  constraint concentric A2 A3
  measures "d9" diameter of A2
  measures "d12" distance of A2 A3
extrude "Extrude3" add sketch "Sketch3" along normal blind 3.6 contours A2
ref_plane "WorkPlane1" through (0, 0, 20) normal (0, 0, -1) x (-1, 0, 0)
sketch "Sketch4" plane through (0, 0, 20) normal (0, 0, -1) x (-1, 0, 0)
  line L0 (-11.5, 6) -> (-15.8, 6)
  line L1 (-15.8, 6) -> (-15.8, -6)
  line L2 (-15.8, -6) -> (-11.5, -6)
  line L3 (-11.5, -6) -> (-11.5, 6)
  circle A0 centre (-14.45, 0) radius 1.5
  point P0 (-11.5, 6)
  point P1 (-11.5, -6)
  dimension "d14" = 4.3
  dimension "d15" = 3
  dimension "d16" = 1.35
  constraint horizontal L0
  constraint vertical L1
  constraint horizontal L2
  constraint vertical L3
  constraint coincident P0 L0.start
  constraint coincident P1 L2.end
  constraint horizontal origin A0.centre
  measures "d14" distance of P0 L0.end
  measures "d15" diameter of A0
  measures "d16" distance of L1 A0.centre
extrude "Extrude4" add sketch "Sketch4" along normal blind 2.3 contours L0 L1 L2 L3 A0
mirror "Mirror1" about plane through (0, 0, 0) normal (1, 0, 0) of "Extrude4"
fillet "Fillet1" radius 0.5 12 edges at (-11.5, -6, 8.85) (-11.5, 6, 8.85) (11.5, -6, 8.85) (11.5, 6, 8.85) (11.5, 6, 22.05) (11.5, -6, 22.05) (-11.5, -6, 22.05) (-11.5, 6, 22.05) (-15.8, -6, 18.85) (-15.8, 6, 18.85) (15.8, -6, 18.85) (15.8, 6, 18.85)

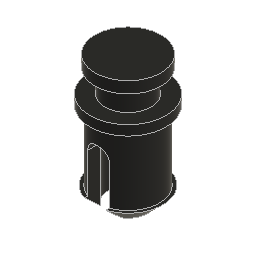
design "Rivet"
Autodesk Fusion 360 part; units mm, degrees
sketch "Sketch1" plane through (0, 0, 0) normal (0, 1, 0) x (1, 0, 0)
  line L0 (0, -7.9) -> (2, -7.9)
  line L1 (2, -7.9) -> (2, -7.2)
  line L2 (2, -7.2) -> (1.4, -7.2)
  line L3 (1.4, -7.2) -> (1.4, -5.8)
  line L4 (1.4, -5.8) -> (2.3, -5.8)
  line L5 (2.3, -5.8) -> (2.3, -5.2)
  line L6 (2.3, -5.2) -> (1.9, -5.2)
  line L7 (1.9, -5.2) -> (1.9, -1)
  line L8 (1.9, -1) -> (2.1, -1)
  line L9 (2.1, -1) -> (1.1, 0)
  line L10 (1.1, 0) -> (0, 0)
  line L11 (0, 0) -> (0, -7.9)
  dimension "d1" = 2
  dimension "d2" = 0.7
  dimension "d3" = 1.4
  dimension "d4" = 1.4
  dimension "d5" = 0.6
  dimension "d6" = 0.4
  dimension "d7" = 1.9
  dimension "d8" = 5.8
  dimension "d9" = 1
  dimension "d10" = 2.1
  dimension "d11" = 135
  constraint horizontal L0
  constraint perpendicular L0 L1
  constraint perpendicular L1 L2
  constraint perpendicular L2 L3
  constraint perpendicular L3 L4
  constraint perpendicular L4 L5
  constraint perpendicular L5 L6
  constraint perpendicular L6 L7
  constraint perpendicular L5 L8
  constraint coincident L10.end L11.start
  constraint parallel L8 L10
  constraint perpendicular L0 L11
  measures "d1" distance of L0.start L0.end
  measures "d2" distance of L0.end L1.end
  measures "d3" distance of L3 L11
  measures "d4" distance of L2.end L3.end
  measures "d5" distance of L4.end L5.end
  measures "d6" distance of L5.end L6.end
  measures "d7" distance of L7 L11
  measures "d8" distance of L4 L10
  measures "d9" distance of L8 L10
  measures "d10" distance of L8.end L11
  measures "d11" angle of L9 L10
revolve "Revolve1" add sketch "Sketch1" angle 360 about axis through (0, 0, 0) along (0, 0, 1)
sketch "Sketch2" plane through (0, 0, 0) normal (0, 0, -1) x (1, 0, 0)
  circle A0 centre (0, 0) radius 1.1
  circle A1 centre (0, 0) radius 1.2
  circle A2 centre (0, 0) radius 2.1
  dimension "d14" = 0.9
  constraint coincident A0.centre A1.centre
  measures "d14" distance of A1 A2
extrude "Extrude1" cut sketch "Sketch2" against normal up to surface (5.2 mm away) contours A0 | A1
sketch "Sketch3" plane through (0, 0, 0) normal (0, 1, 0) x (1, 0, 0)
  line L0 (0.65, 0) -> (0.65, -3.4)
  line L1 (0.65, -3.4) -> (-0.65, -3.4)
  line L2 (-0.65, -3.4) -> (-0.65, 0)
  line L3 (-0.65, 0) -> (0.65, 0)
  circle A0 centre (0, -3.4) radius 0.65
  line L4 (-1.2, -0.1) -> (1.2, -0.1)
  dimension "d17" = 1.3
  dimension "d18" = 0.65
  dimension "d20" = 3.3
  constraint vertical L0
  constraint perpendicular L0 L1
  constraint perpendicular L1 L2
  constraint perpendicular L0 L3
  constraint midpoint L1 A0.centre
  constraint coincident L0.end A0
  constraint coincident origin L3
  measures "d17" distance of L0.start L2.end
  measures "d18" distance of origin L0
  measures "d20" distance of A0.centre L4
extrude "Extrude2" cut sketch "Sketch3" along normal mid plane 6 contours L0 L2 A0 L4 | L1 A0 | L1 A0

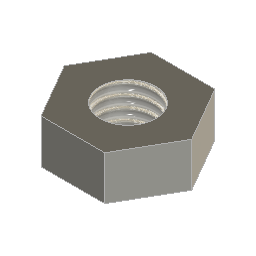
design "M3_nut"
Autodesk Fusion 360 part; units mm, degrees
sketch "Sketch1" plane through (0, 0, 0) normal (0, 0, 1) x (1, 0, 0)
  line L0 (2.8868, 0) -> (1.4434, 2.5)
  line L1 (1.4434, 2.5) -> (-1.4434, 2.5)
  line L2 (-1.4434, 2.5) -> (-2.8868, 0)
  line L3 (-2.8868, 0) -> (-1.4434, -2.5)
  line L4 (-1.4434, -2.5) -> (1.4434, -2.5)
  line L5 (1.4434, -2.5) -> (2.8868, 0)
  circle A0 centre (0, 0) radius 1.5
  dimension "d1" = 5
  dimension "d2" = 3
  constraint coincident A0.centre origin
  constraint horizontal L1
  measures "d1" distance of L0 L3
  measures "d2" diameter of A0
extrude "Extrude1" add sketch "Sketch1" along normal blind 2
thread "Thread1" "ISO Metric profile 3.0 M3x0.5 M3x0.5 6H" major diameter 3.086 minor diameter 2.529 pitch 0.5 angle 60 resizes the face on face at (1.4981, -0.0748, 1.3333)

design "M2.5_nut"
Autodesk Fusion 360 part; units mm, degrees
sketch "Sketch1" plane through (0, 0, 0) normal (0, 0, 1) x (1, 0, 0)
  line L0 (2.0785, 0) -> (1.0392, 1.8)
  line L1 (1.0392, 1.8) -> (-1.0392, 1.8)
  line L2 (-1.0392, 1.8) -> (-2.0785, 0)
  line L3 (-2.0785, 0) -> (-1.0392, -1.8)
  line L4 (-1.0392, -1.8) -> (1.0392, -1.8)
  line L5 (1.0392, -1.8) -> (2.0785, 0)
  circle A0 centre (0, 0) radius 1
  dimension "d1" = 3.6
  dimension "d2" = 2
  constraint coincident A0.centre origin
  constraint horizontal L1
  measures "d1" distance of L0 L3
  measures "d2" diameter of A0
extrude "Extrude1" add sketch "Sketch1" along normal blind 1.5
thread "Thread1" "ISO Metric profile 2.5 M2.5x0.45 M2.5x0.45 6H" major diameter 2.58 minor diameter 2.0755 pitch 0.45 angle 60 resizes the face on face at (0.9988, -0.0498, 1)

design "Servo Mount"
Autodesk Fusion 360 part; units mm, degrees
sketch "Sketch1" plane through (0, 0, 0) normal (0, 0, 1) x (1, 0, 0)
  line L0 (11.55, 6.05) -> (-11.55, 6.05)
  line L1 (-11.55, 6.05) -> (-11.55, -6.05)
  line L2 (-11.55, -6.05) -> (11.55, -6.05)
  line L3 (11.55, -6.05) -> (11.55, 6.05)
  line L4 (11.55, 6.05) -> (-11.55, -6.05) construction
  line L5 (-11.55, 6.05) -> (11.55, -6.05) construction
  line L6 (13.55, -11.05) -> (-13.55, -11.05)
  line L7 (-16.55, -8.05) -> (-16.55, 8.05)
  line L8 (-13.55, 11.05) -> (13.55, 11.05)
  line L9 (16.55, -7) -> (16.55, -8.05)
  line L10 (16.55, -11.05) -> (-16.55, 11.05) construction
  line L11 (-16.55, -11.05) -> (16.55, 11.05) construction
  arc A0 (-13.55, 11.05) -> (-16.55, 8.05) centre (-13.55, 8.05) ccw
  arc A1 (-16.55, -8.05) -> (-13.55, -11.05) centre (-13.55, -8.05) ccw
  arc A2 (13.55, -11.05) -> (16.55, -8.05) centre (13.55, -8.05) ccw
  arc A3 (16.55, 8.05) -> (13.55, 11.05) centre (13.55, 8.05) ccw
  line L12 (18.55, 5) -> (29.55, 5)
  line L13 (31.55, 3) -> (31.55, -3)
  line L14 (29.55, -5) -> (18.55, -5)
  circle A4 centre (21.55, 0) radius 2.5
  arc A5 (29.55, -5) -> (31.55, -3) centre (29.55, -3) ccw
  arc A6 (31.55, 3) -> (29.55, 5) centre (29.55, 3) ccw
  arc A7 (18.55, -5) -> (16.55, -7) centre (18.55, -7) ccw
  line L15 (16.55, 7) -> (16.55, 8.05)
  arc A8 (16.55, 7) -> (18.55, 5) centre (18.55, 7) ccw
  line L16 (0, 0) -> (0, 11.05) construction
  arc A9 (-18.55, 5) -> (-16.55, 7) centre (-18.55, 7) ccw
  arc A10 (-29.55, 5) -> (-31.55, 3) centre (-29.55, 3) ccw
  line L17 (-31.55, 3) -> (-31.55, -3)
  arc A11 (-31.55, -3) -> (-29.55, -5) centre (-29.55, -3) ccw
  line L18 (-29.55, -5) -> (-18.55, -5)
  arc A12 (-16.55, -7) -> (-18.55, -5) centre (-18.55, -7) ccw
  circle A13 centre (-21.55, 0) radius 2.5
  line L19 (-29.55, 5) -> (-18.55, 5)
  circle A14 centre (27.55, 0) radius 2.5
  line L20 (27.55, -2.5) -> (21.55, -2.5)
  line L21 (27.55, 2.5) -> (21.55, 2.5)
  line L22 (-27.55, 2.5) -> (-21.55, 2.5)
  line L23 (-27.55, -2.5) -> (-21.55, -2.5)
  circle A15 centre (-27.55, 0) radius 2.5
  point P0 (16.55, 5)
  point P1 (31.55, 5)
  point P2 (31.55, -5)
  dimension "d1" = 23.1
  dimension "d2" = 12.1
  dimension "d3" = 5
  dimension "d4" = 5
  dimension "d5" = 3
  dimension "d7" = 10
  dimension "d8" = 5
  dimension "d9" = 5
  dimension "d10" = 5
  dimension "d11" = 5
  dimension "d12" = 2
  dimension "d13" = 2
  dimension "d20" = 15
  dimension "d21" = 5
  dimension "d22" = 4
  constraint horizontal L0
  constraint perpendicular L0 L1
  constraint parallel L0 L2
  constraint parallel L1 L3
  constraint coincident L4 L16.start
  constraint coincident L5 L16.start
  constraint coincident L16.start origin
  constraint horizontal L6
  constraint perpendicular L6 L7
  constraint parallel L6 L8
  constraint parallel L7 L9
  constraint coincident L10 L16.start
  constraint coincident L11 L16.start
  constraint coincident L10.end L8
  constraint coincident L10.end L7
  constraint tangent L8 A0
  constraint tangent L7 A0
  constraint coincident L11.start L7
  constraint coincident L11.start L6
  constraint tangent L7 A1
  constraint tangent L6 A1
  constraint equal A0 A1
  constraint coincident L10.start L6
  constraint coincident L10.start L9
  constraint tangent L6 A2
  constraint tangent L9 A2
  constraint equal A0 A2
  constraint coincident L11.end L8
  constraint coincident L11.end L9
  constraint tangent L8 A3
  constraint tangent L9 A3
  constraint equal A0 A3
  constraint coincident L9 P0
  constraint perpendicular L9 L12
  constraint perpendicular L12 L13
  constraint perpendicular L9 L14
  constraint coincident P2 L13
  constraint coincident P2 L14
  constraint tangent L13 A5
  constraint tangent L14 A5
  constraint coincident P1 L12
  constraint coincident P1 L13
  constraint tangent L12 A6
  constraint tangent L13 A6
  constraint equal A5 A6
  constraint coincident L9 A3.start
  constraint tangent L14 A7
  constraint tangent L9 A7
  constraint equal A5 A7
  constraint coincident P0 L15
  constraint coincident P0 L12
  constraint tangent L15 A8
  constraint tangent L12 A8
  constraint midpoint L8 L16.end
  constraint symmetric A4 L16 A13
  constraint symmetric L13.end L16 L17.end
  constraint symmetric L14.start L16 A11.end
  constraint symmetric A5 L16 A11
  constraint symmetric L12.end L16 A10.start
  constraint symmetric L13.start L16 A10.end
  constraint symmetric A6 L16 A10
  constraint symmetric L14.end L16 L18.end
  constraint symmetric L9.start L16 A12.start
  constraint symmetric A7 L16 A12
  constraint symmetric L15.start L16 A9.end
  constraint symmetric L12.start L16 A9.start
  constraint symmetric A8 L16 A9
  constraint horizontal A4.centre A14.centre
  constraint coincident A14 L20.start
  constraint coincident A4 L20.end
  constraint tangent A4 L20
  constraint horizontal L20
  constraint coincident A14 L21.start
  constraint coincident A4 L21.end
  constraint tangent A4 L21
  constraint parallel L12 L21
  constraint symmetric L16 A14 A15
  constraint symmetric L16 L20.start L23.start
  constraint symmetric L16 L20.end L23.end
  constraint symmetric L16 L21.start L22.start
  constraint symmetric L16 L21.end L22.end
  measures "d1" distance of L0.start L0.end
  measures "d2" distance of L0.start L2.end
  measures "d3" distance of L0 L8
  measures "d4" distance of L3 L9
  measures "d5" radius of A0
  measures "d7" distance of P1 P2
  measures "d8" distance of L16.start L12
  measures "d9" diameter of A4
  measures "d10" distance of L9 A4.centre
  measures "d11" distance of L12 A4.centre
  measures "d12" radius of A5
  measures "d13" radius of A8
  measures "d20" distance of L9.end L13
  measures "d21" diameter of A14
  measures "d22" distance of L13 A14.centre
extrude "Extrude1" add sketch "Sketch1" along normal blind 5
sketch "Sketch2" plane through (0, 0, 5) normal (0, 0, 1) x (-1, 0, 0)
  line L0 (-11.55, -6.05) -> (-11.55, 6.05)
  line L1 (-11.55, 6.05) -> (11.55, 6.05)
  line L2 (11.55, 6.05) -> (11.55, -6.05)
  line L3 (11.55, -6.05) -> (-11.55, -6.05)
  line L4 (31.55, -3) -> (31.55, 3)
  arc A0 (31.55, 3) -> (29.55, 5) centre (29.55, 3) ccw
  line L5 (29.55, 5) -> (18.55, 5)
  arc A1 (16.55, 7) -> (18.55, 5) centre (18.55, 7) ccw
  line L6 (16.55, 7) -> (16.55, 8.05)
  arc A2 (16.55, 8.05) -> (13.55, 11.05) centre (13.55, 8.05) ccw
  line L7 (13.55, 11.05) -> (-13.55, 11.05)
  arc A3 (-13.55, 11.05) -> (-16.55, 8.05) centre (-13.55, 8.05) ccw
  line L8 (-16.55, 8.05) -> (-16.55, 7)
  arc A4 (-18.55, 5) -> (-16.55, 7) centre (-18.55, 7) ccw
  line L9 (-18.55, 5) -> (-29.55, 5)
  arc A5 (-29.55, 5) -> (-31.55, 3) centre (-29.55, 3) ccw
  line L10 (-31.55, 3) -> (-31.55, -3)
  arc A6 (-31.55, -3) -> (-29.55, -5) centre (-29.55, -3) ccw
  line L11 (-29.55, -5) -> (-18.55, -5)
  arc A7 (-16.55, -7) -> (-18.55, -5) centre (-18.55, -7) ccw
  line L12 (-16.55, -7) -> (-16.55, -8.05)
  arc A8 (-16.55, -8.05) -> (-13.55, -11.05) centre (-13.55, -8.05) ccw
  line L13 (-13.55, -11.05) -> (13.55, -11.05)
  arc A9 (13.55, -11.05) -> (16.55, -8.05) centre (13.55, -8.05) ccw
  line L14 (16.55, -8.05) -> (16.55, -7)
  arc A10 (18.55, -5) -> (16.55, -7) centre (18.55, -7) ccw
  line L15 (18.55, -5) -> (29.55, -5)
  arc A11 (29.55, -5) -> (31.55, -3) centre (29.55, -3) ccw
  circle A12 centre (-14.5, 0) radius 1.5
  line L16 (0, 0) -> (0, 6.05) construction
  circle A13 centre (14.5, 0) radius 1.5
  line L17 (21.55, 2.5) -> (27.55, 2.5)
  arc A14 (27.55, -2.5) -> (27.55, 2.5) centre (27.55, 0) ccw
  line L18 (27.55, -2.5) -> (21.55, -2.5)
  arc A15 (21.55, 2.5) -> (21.55, -2.5) centre (21.55, 0) ccw
  arc A16 (-27.55, 2.5) -> (-27.55, -2.5) centre (-27.55, 0) ccw
  line L19 (-27.55, 2.5) -> (-21.55, 2.5)
  arc A17 (-21.55, -2.5) -> (-21.55, 2.5) centre (-21.55, 0) ccw
  line L20 (-21.55, -2.5) -> (-27.55, -2.5)
  dimension "d16" = 3
  dimension "d17" = 2.95
  constraint horizontal L16.start A12.centre
  constraint coincident L16.start origin
  constraint midpoint L1 L16.end
  constraint symmetric A12 L16 A13
  measures "d16" diameter of A12
  measures "d17" distance of L0 A12.centre
extrude "Extrude2" add sketch "Sketch2" along normal blind 20 draft -0.8 contours A12 | A13

design "Motor Mount"
Autodesk Fusion 360 part; units mm, degrees